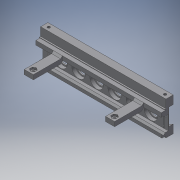
# Autodesk Inventor part: Case_top_back
Saved by Autodesk Inventor 2016 SP2 (Build 200236200, 236)
## iProperties
Created: 2018-06-26
Part Number: Case_top_back
Material: Generisch
Document SubType Name: Modeling
Designer: Nils
Density: 1 g/cm^3
Appearance: Vorgabe
Author: Nils
Autodesk Inventor part; units mm, degrees
ref_plane "YZ Plane" through (0, 0, 0) normal (1, 0, 0) x (0, 1, 0)
ref_plane "XZ Plane" through (0, 0, 0) normal (0, 1, 0) x (-1, 0, 0)
ref_plane "XY Plane" through (0, 0, 0) normal (0, 0, 1) x (1, 0, 0)
sketch "Skizze1" plane through (0, 0, 0) normal (1, 0, 0) x (0, 1, 0)
  line L0 (14.121, 246.6563) -> (22.121, 246.6563) projected
  line L1 (14.121, 237.3563) -> (14.121, 246.6563) projected
  line L2 (22.121, 246.6563) -> (22.121, 237.2328) projected
  line L3 (22.121, 218.7798) -> (22.121, 209.3563) projected
  line L4 (22.121, 209.3563) -> (14.121, 209.3563) projected
  line L5 (14.121, 214.8563) -> (14.121, 209.3563) projected
  line L6 (12.621, 237.3563) -> (14.121, 237.3563) projected
  line L7 (12.621, 237.3563) -> (12.621, 236.8563) projected
  line L8 (13.371, 236.1063) -> (12.621, 236.8563) projected
  line L9 (22.121, 237.2328) -> (22.121, 218.7798)
  line L10 (14.121, 209.3563) -> (14.121, 211.3563)
  line L11 (14.121, 211.3563) -> (9.621, 211.3563)
  line L12 (9.621, 211.3563) -> (9.621, 214.8563)
  line L13 (9.621, 214.8563) -> (11.421, 213.0563)
  line L14 (11.421, 213.0563) -> (13.221, 214.8563)
  line L15 (13.221, 214.8563) -> (16.691, 214.8563)
  line L16 (16.691, 214.8563) -> (16.691, 230.8263)
  line L17 (16.691, 230.8263) -> (11.721, 230.8263)
  line L18 (11.721, 230.8263) -> (9.921, 232.6263)
  line L19 (11.721, 230.8263) -> (14.2666, 230.8263) construction
  line L20 (9.921, 232.6263) -> (8.871, 231.5763)
  line L21 (8.871, 231.5763) -> (8.871, 236.1063)
  line L22 (8.871, 236.1063) -> (13.371, 236.1063)
  point P0 (0, 0)
  dimension "d0" = 2
  dimension "d1" = 4.5
  dimension "d2" = 3.5
  dimension "d3" = 3.47
  dimension "d4" = 15.97
  dimension "d5" = 1.8
  dimension "d6" = 45
  dimension "d7" = 135
  dimension "d8" = 4.53
  dimension "d9" = 1.8
  dimension "d10" = 4.5
  dimension "d71" = 5.43
  constraints: 28 end point, 7 perpendicular, 2 equal length, 2 vertical, 1 horizontal, 1 parallel, 1 point on line
  measures "d0" distance of L4.end L10.end
  measures "d1" distance of L10.end L11.end
  measures "d2" distance of L11.end L12.end
  measures "d3" distance of L14.end L15.end
  measures "d4" distance of L15.end L16.end
  measures "d5" horizontal distance of L12.end L13.end
  measures "d6" angle of L13 L12
  measures "d7" angle of L19 L18
  measures "d8" distance of L20.end L21.end
  measures "d9" horizontal distance of L18.end L17.end
  measures "d10" distance of L21.end L8.start
  measures "d71" distance between parallel lines of L3 L16
extrude "Extrusion1" add sketch "Skizze1" along normal blind 69.4
sketch "Skizze2" plane through (0, 22.121, 246.6563) normal (0, 1, 0) x (1, 0, 0)
  line L0 (0, 0) -> (138.8, 0) projected
  line L1 (10.1, 3.4768) -> (10.1, 33.8232) projected
  line L2 (0, 37.3) -> (138.8, 37.3) projected
  line L3 (0, 9.308) -> (0, 27.992)
  line L4 (0, 37.3) -> (0, 0) projected
  line L5 (0, 0) -> (0, 9.308) projected
  line L6 (0, 9.308) -> (10.1, 3.4768) projected
  line L7 (10.1, 33.8232) -> (0, 27.992) projected
  line L8 (0, 27.992) -> (0, 37.3) projected
  line L9 (138.8, 27.992) -> (128.7, 33.8232) projected
  line L10 (128.7, 33.8232) -> (128.7, 3.4768) projected
  line L11 (128.7, 3.4768) -> (138.8, 9.308) projected
  line L12 (138.8, 0) -> (138.8, 9.308) projected
  line L13 (138.8, 27.992) -> (138.8, 37.3) projected
  point P0 (0, 246.6563)
  constraints: 2 end point, 1 collinear
extrude "Extrusion2" cut sketch "Skizze2" against normal blind 5 contours L3 L7 L1 L6
sketch "Skizze3" plane through (0, 8.871, 231.5763) normal (0, -1, 0) x (1, 0, 0)
  line L0 (19.4, 2.53) -> (29.4, 2.53) projected
  line L1 (29.4, 2.53) -> (29.4, -2.47) projected
  line L2 (29.4, -2.47) -> (19.4, -2.47) projected
  line L3 (19.4, -2.47) -> (19.4, 2.53) projected
  point P0 (0, -231.5763)
extrude "Extrusion3" add sketch "Skizze3" along normal blind 32.25
chamfer "Fase1" distance 2.4 angle 45 1 edges at (24.4, 8.871, 229.1063)
chamfer "Fase2" distance 2 angle 45 1 edges at (24.4, 8.871, 234.1063)
sketch "Skizze4" plane through (29.4, -23.379, 229.1063) normal (0, 0, -1) x (-1, 0, 0)
  circle A0 centre (5, 5) radius 1.75
  line L0 (0, 0) -> (10, 0) projected
  line L1 (10, 30.25) -> (10, 0) projected
  point P0 (29.4, 23.379)
  point P1 (10, 32.25)
  dimension "d23" = 3.5
  dimension "d24" = 5
  dimension "d25" = 5
  constraints: 1 centre point
  measures "d23" diameter of A0
  measures "d24" distance from line of L0 A0.centre
  measures "d25" distance from line of L1 A0.centre
extrude "Extrusion4" cut sketch "Skizze4" against normal blind 32.25
sketch "Skizze6" plane through (0, 14.121, 246.6563) normal (0, 0, 1) x (1, 0, 0)
  circle A0 centre (5, 4) radius 1.5 projected
extrude "Extrusion5" cut sketch "Skizze6" against normal blind 34.75
sketch "Skizze7" plane through (0, 8.871, 231.5763) normal (0, -1, 0) x (1, 0, 0)
  line L0 (7.85, -2.17) -> (2.15, -2.17) projected
  line L1 (7.85, -4.97) -> (7.85, -2.17) projected
  line L2 (2.15, -4.97) -> (7.85, -4.97) projected
  line L3 (2.15, -2.17) -> (2.15, -4.97) projected
  point P0 (0, -231.5763)
extrude "Extrusion6" cut sketch "Skizze7" against normal blind 11.25
mirror "Spiegeln1" about plane through (69.4, 16.7548, 227.0605) normal (1, 0, 0) of "Extrusion6", "Extrusion5", "Extrusion4", "Extrusion3", "Extrusion2", "Extrusion1", "Fase2", "Fase1"
sketch "Skizze10" plane through (19.4, -23.379, 234.1063) normal (0, 0, 1) x (1, 0, 0)
  circle A0 centre (5, 5) radius 1.75 construction
  circle A1 centre (95, 5) radius 1.75 construction
  line L0 (2.15, 6.6454) -> (5, 8.2909)
  line L1 (5, 8.2909) -> (7.85, 6.6454)
  line L2 (7.85, 6.6454) -> (7.85, 3.3546)
  line L3 (7.85, 3.3546) -> (5, 1.7091)
  line L4 (5, 1.7091) -> (2.15, 3.3546)
  line L5 (2.15, 3.3546) -> (2.15, 6.6454)
  circle A2 centre (95, 5) radius 1.75 projected
  line L6 (92.15, 6.6454) -> (95, 8.2909)
  line L7 (95, 8.2909) -> (97.85, 6.6454)
  line L8 (97.85, 6.6454) -> (97.85, 3.3546)
  line L9 (97.85, 3.3546) -> (95, 1.7091)
  line L10 (95, 1.7091) -> (92.15, 3.3546)
  line L11 (92.15, 3.3546) -> (92.15, 6.6454)
  point P0 (-19.4, 23.379)
  dimension "d51" = 5.7
  dimension "d52" = 5.7
  constraints: 24 end point, 2 coincident, 2 vertical, 26 other
  measures "d51" distance between parallel lines of L2 L5
  measures "d52" distance between parallel lines of L8 L11
extrude "Extrusion9" cut sketch "Skizze10" against normal blind 2.2
sketch "Skizze11" plane through (0, 22.121, 246.6563) normal (0, 1, 0) x (1, 0, 0)
  line L0 (138.8, 15.83) -> (138.8, 31.8) construction
  line L1 (0, 15.83) -> (0, 31.8) construction
  line L2 (138.8, 23.815) -> (0, 23.815) construction
  circle A0 centre (119.4, 23.815) radius 6
  dimension "d61" = 12
  dimension "d62" = 19.4
  constraints: 2 end point, 2 midpoint, 1 centre point, 1 point on line
  measures "d61" diameter of A0
  measures "d62" distance from line of L0 A0.centre
extrude "Extrusion10" cut sketch "Skizze11" against normal blind 5.5
sketch "Skizze12" plane through (6.0088, 16.691, -38.3137) normal (0, -1, 0) x (1, 0, 0)
  circle A0 centre (113.3912, 261.155) radius 6 construction
  circle A1 centre (113.3912, 261.155) radius 7.5
  point P0 (-6.0088, 38.3137)
  dimension "d65" = 15
  constraints: 1 centre point, 1 coincident
  measures "d65" diameter of A1
extrude "Extrusion11" cut sketch "Skizze12" against normal blind 4
pattern_linear "Rechteckige Anordnung1" count 6 spacing 20 along (-1, 0, 0) of "Extrusion11", "Extrusion10"
